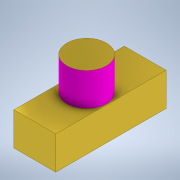
# Autodesk Inventor part: mass applied
Saved by Autodesk Inventor 2021 (Build 250183000, 183)
## iProperties
Created: 2021-07-28
Part Number: mass applied
Material: Iron, Cast
Document SubType Name: Modeling
Designer: Shammy Haider
Mass: 38.0016 g
Surface Area: 21.3245 cm^2
Volume: 5.31491 cm^3
Density: 7.15 g/cm^3
Appearance: Metal 2400F Hot
Author: Shammy Haider
Autodesk Inventor part; units mm, degrees
ref_plane "YZ Plane" through (0, 0, 0) normal (1, 0, 0) x (0, 1, 0)
ref_plane "XZ Plane" through (0, 0, 0) normal (0, 1, 0) x (-1, 0, 0)
ref_plane "XY Plane" through (0, 0, 0) normal (0, 0, 1) x (1, 0, 0)
sketch "Sketch1" plane through (0, 0, 0) normal (0, 1, 0) x (-1, 0, 0)
  line L0 (12.6229, 24.94) -> (0, 24.94)
  line L1 (0, 24.94) -> (0, -8.3425)
  line L2 (0, -8.3425) -> (12.6229, -8.3425)
  line L3 (12.6229, -8.3425) -> (12.6229, 24.94)
  line L4 (12.6229, 24.94) -> (0, -8.3425) construction
  line L5 (0, 24.94) -> (12.6229, -8.3425) construction
  point P0 (0, 0)
  point P1 (6.3114, 8.2988)
  constraints: 12 end point, 2 midpoint, 2 parallel, 1 horizontal, 1 perpendicular
extrude "Extrusion1" add sketch "Sketch1" along normal blind 10
sketch "Sketch2" plane through (0, 10, 0) normal (0, 1, 0) x (1, 0, 0)
  circle A0 centre (-6.1347, -9.4794) radius 5.954
  point P0 (0, 0)
  constraints: 1 centre point
extrude "Extrusion2" add sketch "Sketch2" along normal blind 10
body "Solid1"
